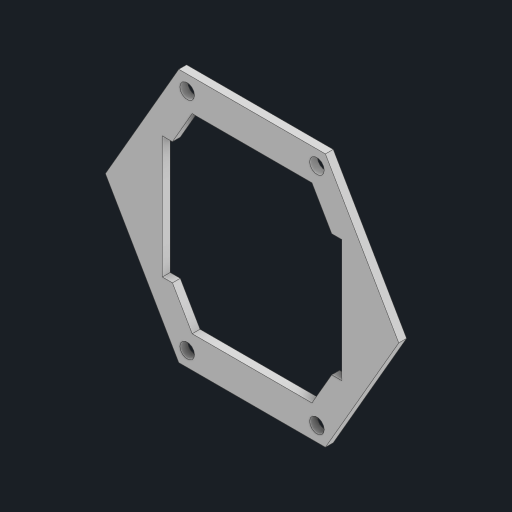
# Autodesk Inventor part: ArmDriverBoard
Saved by Autodesk Inventor 2023 (Build 270158000, 158)
## iProperties
Created: 2023-12-27
Part Number: ArmDriverBoard
Material: Generic
Document SubType Name: Sheet Metal
Designer: valer
Density: 1 g/cm^3
Sheet Metal Rule: Default_mm
Appearance: Default
Author: valer
Autodesk Inventor part; units mm, degrees
ref_plane "YZ Plane" through (0, 0, 0) normal (1, 0, 0) x (0, 1, 0)
ref_plane "XZ Plane" through (0, 0, 0) normal (0, 1, 0) x (-1, 0, 0)
ref_plane "XY Plane" through (0, 0, 0) normal (0, 0, 1) x (1, 0, 0)
sketch "Base" plane through (0, 0, 0) normal (0, 0, 1) x (1, 0, 0)
  line L0 (-12.251, -19.5001) -> (-16.2925, -12.5001)
  line L1 (-16.2925, -12.5001) -> (-18.35, -12.5001)
  line L2 (-18.35, -12.5001) -> (-18.35, 12.5)
  line L3 (-18.35, 12.5) -> (-16.2925, 12.5)
  line L4 (-16.2925, 12.5) -> (-12.251, 19.5)
  line L5 (15, 25.9807) -> (-15, 25.9807)
  line L6 (-15, 25.9807) -> (-30, 0)
  line L7 (-30, 0) -> (-15, -25.9808)
  line L8 (-15, -25.9808) -> (15, -25.9808)
  line L9 (15, -25.9808) -> (30, 0)
  line L10 (30, 0) -> (15, 25.9807)
  circle A0 centre (-13.2679, 22.9807) radius 1.5
  line L11 (-42, 0) -> (42, 0) construction
  line L12 (0, -36.3731) -> (0, 36.373) construction
  circle A1 centre (13.2679, 22.9807) radius 1.5
  circle A2 centre (-13.2679, -22.9807) radius 1.5
  circle A3 centre (13.2679, -22.9807) radius 1.5
  line L13 (-12.251, 19.5) -> (0, 19.5)
  line L14 (-12.251, -19.5001) -> (0, -19.5001)
  line L15 (18.35, 12.5) -> (16.2925, 12.5)
  line L16 (12.251, -19.5001) -> (16.2925, -12.5001)
  line L17 (18.35, -12.5001) -> (18.35, 12.5)
  line L18 (16.2925, 12.5) -> (12.251, 19.5)
  line L19 (16.2925, -12.5001) -> (18.35, -12.5001)
  line L20 (12.251, 19.5) -> (0, 19.5)
  line L21 (12.251, -19.5001) -> (0, -19.5001)
  point P0 (0, 0)
  point P1 (0, 0)
  point P2 (0, 25.9807)
  dimension "d0" = 30
  dimension "d1" = 30
  dimension "d2" = 120
  dimension "d3" = 120
  dimension "d4" = 120
  dimension "d5" = 120
  dimension "d6" = 3
  dimension "d7" = 3
  dimension "d8" = 3
  dimension "d10" = 18.35
  dimension "d13" = 2.0575
  dimension "d14" = 6.4807
  dimension "d15" = 6.4807
  dimension "d16" = 25.0001
  dimension "d17" = 22.9807
  dimension "d18" = 7
  measures "d0" distance of L10.end L6.start
  measures "d1" distance of L9.end L10.end
  measures "d2" angle of L10 L5
  measures "d3" angle of L5 L6
  measures "d4" angle of L8 L7
  measures "d5" angle of L9 L8
  measures "d6" distance from line of L5 A0.centre
  measures "d7" distance from line of L6 A0.centre
  measures "d8" diameter of A0
  measures "d10" distance between parallel lines of L12 L2
  measures "d13" distance of L3.start L3.end
  measures "d14" distance from line of L5 L4.end
  measures "d15" distance from line of L8 L0.start
  measures "d16" distance of L2.start L3.start
  measures "d18" vertical distance of L3.end L4.end
extrude "Plate1" add sketch "Base" along normal blind 1.6002
equation "\"d2\" = d3"
equation "\"d4\" = d3"
equation "\"d5\" = d3"
equation "\"d15\" = d14"
equation "\"d19\" = Thickness"
equation "\"BendRadius\" = Thickness"
equation "\"BendReliefWidth\" = Thickness"
equation "\"BendReliefDepth\" = 0.5 * Thickness"
equation "\"CornerReliefSize\" = 4 * Thickness"
equation "\"MinimumRemnant\" = 2 * Thickness"
equation "\"TransitionRadius\" = BendRadius"
equation "\"JacobiRadiusSize\" = BendRadius"
equation "\"GapSize\" = Thickness"
equation "\"Thickness\" = 1.6002"
body "Solid1"
